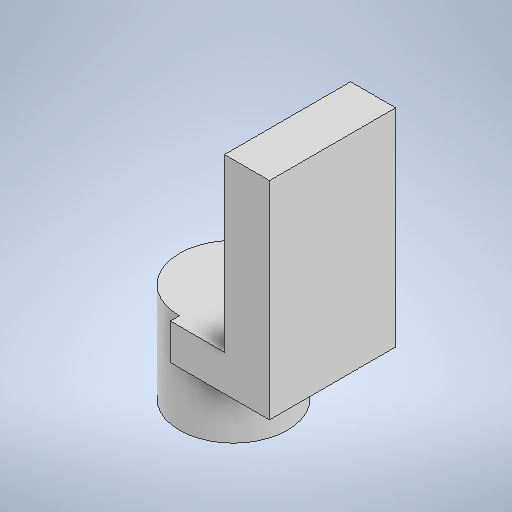
# Autodesk Inventor part: chwytak_rurki
Saved by Autodesk Inventor 2025 (Build 290162000, 162)
## iProperties
Created: 2024-04-14
Part Number: chwytak_rurki
Material: Ogólny
Document SubType Name: Modeling
Designer: user
Density: 1 g/cm^3
Appearance: Domyślna
Author: user
Autodesk Inventor part; units mm, degrees
ref_plane "YZ Plane" through (0, 0, 0) normal (1, 0, 0) x (0, 1, 0)
ref_plane "XZ Plane" through (0, 0, 0) normal (0, 1, 0) x (-1, 0, 0)
ref_plane "XY Plane" through (0, 0, 0) normal (0, 0, 1) x (1, 0, 0)
sketch "Szkic1" plane through (0, 0, 0) normal (0, 1, 0) x (-1, 0, 0)
  circle A0 centre (0, 0) radius 4
  line L0 (0, 7) -> (0, -7)
  line L1 (0, -7) -> (-11, -7)
  line L2 (-11, -7) -> (-11, 7)
  line L3 (-11, 7) -> (0, 7)
  line L4 (-11, 7) -> (-6, 7)
  line L5 (-6, -7) -> (-11, -7)
  line L6 (-11, -7) -> (-11, 7)
  circle A1 centre (0, 0) radius 6
  line L7 (-6, -7) -> (-6, 7)
  point P0 (0, -6)
  point P1 (0, 6)
  point P2 (0, -4)
  point P3 (0, 4)
  point P4 (-6, 0)
  dimension "d0" = 8
  dimension "d1" = 14
  dimension "d2" = 11
  dimension "d3" = 7
  dimension "d6" = 0
  dimension "d7" = 5
  dimension "d8" = 12
  dimension "d15" = 5
  constraints: 16 end point, 3 parallel, 2 centre point, 2 coincident, 2 perpendicular, 1 horizontal, 1 point on line, 1 vertical
  measures "d0" diameter of A0
  measures "d1" distance of L0.start L0.end
  measures "d2" distance of L0.end L1.end
  measures "d3" distance from line of A0.centre L3
  measures "d6" distance from line of point (0, 0) L0
  measures "d7" distance of L5.start L5.end
  measures "d8" diameter of A1
  measures "d15" distance between parallel lines of L2 L7
extrude "Wyciągnięcie proste4" add sketch "Szkic1" against normal blind 10 contours A0 L0 A1 | A0 L0 A1
extrude "Wyciągnięcie proste5" add sketch "Szkic1" along normal mid plane 2 contours A0 L0 | A0 L0 A1 | L0 A0 | A0 L0 A1
extrude "Wyciągnięcie proste6" add sketch "Szkic1" along normal blind 1 contours A1 L7 L3 L0 | L0 L1 L7 A1
extrude "Wyciągnięcie proste7" add sketch "Szkic1" along normal blind 20 contours L7 L1 L2 L3
extrude "Wyciągnięcie proste8" add sketch "Szkic1" against normal blind 3 contours A1 L7 L3 L0 | L0 L1 L7 A1
extrude "Wyciągnięcie proste9" add sketch "Szkic1" against normal blind 3 contours L7 L1 L2 L3
